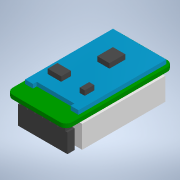
# Autodesk Inventor part: BMS
Saved by Autodesk Inventor 2020 (Build 240168000, 168)
## iProperties
Created: 2021-03-29
Part Number: BMS
Material: Generic
Document SubType Name: Modeling
Designer: Luke
Density: 1 g/cm^3
Appearance: Default
Author: Luke
Autodesk Inventor part; units mm, degrees
ref_plane "YZ Plane" through (0, 0, 0) normal (1, 0, 0) x (0, 1, 0)
ref_plane "XZ Plane" through (0, 0, 0) normal (0, 1, 0) x (-1, 0, 0)
ref_plane "XY Plane" through (0, 0, 0) normal (0, 0, 1) x (1, 0, 0)
sketch "Sketch1" plane through (0, 0, 0) normal (0, 1, 0) x (-1, 0, 0)
  line L0 (7.5, 17.125) -> (-7.5, 17.125)
  line L1 (-9.5, 15.125) -> (-9.5, -15.125)
  line L2 (-7.5, -17.125) -> (7.5, -17.125)
  line L3 (9.5, -15.125) -> (9.5, 15.125)
  line L4 (9.5, 17.125) -> (-9.5, -17.125) construction
  line L5 (-9.5, 17.125) -> (9.5, -17.125) construction
  arc A0 (7.5, -17.125) -> (9.5, -15.125) centre (7.5, -15.125) ccw
  arc A1 (-9.5, -15.125) -> (-7.5, -17.125) centre (-7.5, -15.125) ccw
  arc A2 (-7.5, 17.125) -> (-9.5, 15.125) centre (-7.5, 15.125) ccw
  arc A3 (9.5, 15.125) -> (7.5, 17.125) centre (7.5, 15.125) ccw
  point P0 (0, 0)
  dimension "d0" = 19
  dimension "d1" = 34.25
  dimension "d2" = 2
  constraints: 12 end point, 8 point on circle, 8 point on line, 8 tangent, 4 centre point, 3 equal radius, 2 midpoint, 2 parallel, 1 horizontal, 1 perpendicular
  measures "d0" distance of L5.end L4.end
  measures "d1" distance of L4.end L5.start
  measures "d2" radius of A0
extrude "Extrusion1" add sketch "Sketch1" along normal blind 1.28
sketch "Sketch2" plane through (0, 1.28, 0) normal (0, 1, 0) x (1, 0, 0)
  line L0 (8.5, -12.175) -> (8.5, 15.825)
  line L1 (8.5, 15.825) -> (-8.5, 15.825)
  line L2 (-8.5, 15.825) -> (-8.5, -12.175)
  line L3 (-8.5, -12.175) -> (8.5, 15.825) construction
  line L4 (8.5, -12.175) -> (-8.5, 15.825) construction
  line L5 (7.5, 17.125) -> (-7.5, 17.125) projected
  line L6 (0, 17.125) -> (0, 15.825)
  line L7 (-6, -10.975) -> (6, -10.975)
  line L8 (6, -10.975) -> (6, -12.175)
  line L9 (-6, -12.175) -> (-6, -10.975)
  line L10 (-8.5, -12.175) -> (-6, -12.175)
  line L11 (6, -12.175) -> (8.5, -12.175)
  point P0 (0, 0)
  point P1 (0, 15.825)
  dimension "d5" = 17
  dimension "d6" = 28
  dimension "d7" = 1.3
  dimension "d9" = 1.2
  constraints: 22 end point, 4 parallel, 3 horizontal, 3 perpendicular, 2 midpoint, 1 vertical
  measures "d5" distance of L1.end L0.end
  measures "d6" distance of L0.end L0.start
  measures "d7" distance of L6.start L6.end
  measures "d9" distance of L7.end L8.end
extrude "Extrusion2" add sketch "Sketch2" along normal blind 1.28
sketch "Sketch3" plane through (0, 0, 0) normal (0, -1, 0) x (1, 0, 0)
  line L0 (5.75, -9.895) -> (-5.75, -9.895)
  line L1 (-5.75, -9.895) -> (-5.75, 6.605)
  line L2 (-5.75, 6.605) -> (5.75, 6.605)
  line L3 (5.75, 6.605) -> (5.75, -9.895)
  line L4 (7.5, -17.125) -> (-7.5, -17.125) projected
  line L5 (0, -17.125) -> (0, -9.895)
  point P0 (0, 0)
  point P1 (0, -9.895)
  dimension "d12" = 11.5
  dimension "d13" = 16.5
  dimension "d14" = 7.23
  constraints: 10 end point, 2 midpoint, 2 parallel, 1 horizontal, 1 perpendicular, 1 vertical
  measures "d12" distance of L1.end L2.end
  measures "d13" distance of L0.end L1.end
  measures "d14" distance of L5.start L5.end
extrude "Extrusion3" add sketch "Sketch3" along normal blind 1.28
sketch "Sketch4" plane through (0, 0, 0) normal (0, -1, 0) x (1, 0, 0)
  line L0 (-7.5, 17.125) -> (7.5, 17.125) projected
  line L1 (0, 17.125) -> (0, 15.125)
  line L2 (0.2, 15.125) -> (2.24, 15.125)
  line L3 (2.44, 14.925) -> (2.44, 12.885)
  line L4 (2.24, 12.685) -> (0.2, 12.685)
  line L5 (0, 12.885) -> (0, 14.925)
  line L6 (0, 14.925) -> (0.2, 15.125)
  line L7 (2.24, 15.125) -> (2.44, 14.925)
  line L8 (2.44, 12.885) -> (2.24, 12.685)
  line L9 (0.2, 12.685) -> (0, 12.885)
  line L10 (2.64, 15.125) -> (4.68, 15.125)
  line L11 (4.88, 14.925) -> (4.88, 12.885)
  line L12 (4.68, 12.685) -> (2.64, 12.685)
  line L13 (2.44, 12.885) -> (2.44, 14.925)
  line L14 (2.44, 14.925) -> (2.64, 15.125)
  line L15 (4.68, 15.125) -> (4.88, 14.925)
  line L16 (4.88, 12.885) -> (4.68, 12.685)
  line L17 (2.64, 12.685) -> (2.44, 12.885)
  line L18 (5.08, 15.125) -> (7.12, 15.125)
  line L19 (7.32, 14.925) -> (7.32, 12.885)
  line L20 (7.12, 12.685) -> (5.08, 12.685)
  line L21 (4.88, 12.885) -> (4.88, 14.925)
  line L22 (4.88, 14.925) -> (5.08, 15.125)
  line L23 (7.12, 15.125) -> (7.32, 14.925)
  line L24 (7.32, 12.885) -> (7.12, 12.685)
  line L25 (5.08, 12.685) -> (4.88, 12.885)
  line L26 (-2.24, 15.125) -> (-0.2, 15.125)
  line L27 (0, 14.925) -> (0, 12.885)
  line L28 (-0.2, 12.685) -> (-2.24, 12.685)
  line L29 (-2.44, 12.885) -> (-2.44, 14.925)
  line L30 (-2.44, 14.925) -> (-2.24, 15.125)
  line L31 (-0.2, 15.125) -> (0, 14.925)
  line L32 (0, 12.885) -> (-0.2, 12.685)
  line L33 (-2.24, 12.685) -> (-2.44, 12.885)
  line L34 (-4.68, 15.125) -> (-2.64, 15.125)
  line L35 (-2.44, 14.925) -> (-2.44, 12.885)
  line L36 (-2.64, 12.685) -> (-4.68, 12.685)
  line L37 (-4.88, 12.885) -> (-4.88, 14.925)
  line L38 (-4.88, 14.925) -> (-4.68, 15.125)
  line L39 (-2.64, 15.125) -> (-2.44, 14.925)
  line L40 (-2.44, 12.885) -> (-2.64, 12.685)
  line L41 (-4.68, 12.685) -> (-4.88, 12.885)
  line L42 (-7.12, 15.125) -> (-5.08, 15.125)
  line L43 (-4.88, 14.925) -> (-4.88, 12.885)
  line L44 (-5.08, 12.685) -> (-7.12, 12.685)
  line L45 (-7.32, 12.885) -> (-7.32, 14.925)
  line L46 (-7.32, 14.925) -> (-7.12, 15.125)
  line L47 (-5.08, 15.125) -> (-4.88, 14.925)
  line L48 (-4.88, 12.885) -> (-5.08, 12.685)
  line L49 (-7.12, 12.685) -> (-7.32, 12.885)
  point P0 (0, 0)
  point P1 (2.44, 12.685)
  point P2 (2.44, 15.125)
  point P3 (0, 12.685)
  point P4 (2.44, 15.125)
  point P5 (4.88, 12.685)
  point P6 (4.88, 15.125)
  point P7 (2.44, 12.685)
  point P8 (4.88, 15.125)
  point P9 (7.32, 12.685)
  point P10 (7.32, 15.125)
  point P11 (4.88, 12.685)
  point P12 (-2.44, 15.125)
  point P13 (0, 12.685)
  point P14 (-2.44, 12.685)
  point P15 (-4.88, 15.125)
  point P16 (-2.44, 12.685)
  point P17 (-2.44, 15.125)
  point P18 (-4.88, 12.685)
  point P19 (-7.32, 15.125)
  point P20 (-4.88, 12.685)
  point P21 (-4.88, 15.125)
  point P22 (-7.32, 12.685)
  dimension "d27" = 2
  constraints: 98 end point, 48 point on line, 12 parallel, 6 horizontal, 6 perpendicular, 1 midpoint, 1 vertical
  measures "d27" distance of L1.start L1.end
extrude "Extrusion4" add sketch "Sketch4" along normal blind 2.44
sketch "Sketch5" plane through (0, -2.44, 0) normal (0, -1, 0) x (1, 0, 0)
  line L0 (-7.865, 15.055) -> (7.865, 15.055)
  line L1 (7.865, 15.055) -> (7.865, 12.755)
  line L2 (7.865, 12.755) -> (-7.865, 12.755)
  line L3 (-7.865, 12.755) -> (-7.865, 15.055)
  line L4 (0.2, 12.685) -> (0, 12.885) projected
  line L5 (0, 14.925) -> (0, 12.885)
  point P0 (0, 0)
  point P1 (0, 13.905)
  point P2 (0, 13.905)
  dimension "d30" = 15.73
  dimension "d31" = 2.3
  constraints: 10 end point, 2 parallel, 1 horizontal, 1 midpoint, 1 perpendicular, 1 vertical
  measures "d30" distance of L1.end L2.end
  measures "d31" distance of L0.end L1.end
extrude "Extrusion5" add sketch "Sketch5" along normal blind 6
sketch "Sketch6" plane through (0, 2.56, 0) normal (0, 1, 0) x (1, 0, 0)
  line L0 (-1.9361, 4.2441) -> (1.9639, 4.2441)
  line L1 (1.9639, 4.2441) -> (1.9639, 9.2441)
  line L2 (1.9639, 9.2441) -> (-1.9361, 9.2441)
  line L3 (-1.9361, 9.2441) -> (-1.9361, 4.2441)
  line L4 (-6.3946, -7.0839) -> (-2.0946, -7.0839)
  line L5 (-2.0946, -7.0839) -> (-2.0946, -3.9839)
  line L6 (-2.0946, -3.9839) -> (-6.3946, -3.9839)
  line L7 (-6.3946, -3.9839) -> (-6.3946, -7.0839)
  line L8 (3.9309, -7.1914) -> (5.5309, -7.1914)
  line L9 (5.5309, -7.1914) -> (5.5309, -4.1914)
  line L10 (5.5309, -4.1914) -> (3.9309, -4.1914)
  line L11 (3.9309, -4.1914) -> (3.9309, -7.1914)
  line L12 (8.5, 15.825) -> (-8.5, 15.825) projected
  point P0 (0, 0)
  point P1 (3.9309, -5.6914)
  point P2 (0, 15.825)
  point P3 (0.0139, 9.2441)
  point P4 (-2.0946, -5.5339)
  dimension "d34" = 3.9
  dimension "d35" = 5
  dimension "d36" = 4.3
  dimension "d37" = 3.1
  dimension "d38" = 1.6
  dimension "d39" = 3
  constraints: 24 end point, 6 parallel, 4 midpoint, 3 horizontal, 3 perpendicular
  measures "d34" distance of L2.end L1.end
  measures "d35" distance of L1.end L0.end
  measures "d36" distance of L6.end L5.end
  measures "d37" distance of L5.end L4.end
  measures "d38" distance of L10.end L9.end
  measures "d39" distance of L9.end L8.end
extrude "Extrusion6" add sketch "Sketch6" along normal blind 1.5
sketch "Sketch7" plane through (0, -1.28, 0) normal (0, -1, 0) x (1, 0, 0)
  line L0 (-9, 11.5) -> (9, 11.5)
  line L1 (9, 11.5) -> (9, -11.5)
  line L2 (-8.5, -11.5) -> (-9, -11.5)
  line L3 (-9, -11.5) -> (-9, 11.5)
  line L4 (-9, -11.5) -> (-9, -15)
  line L5 (-8.5, -15.825) -> (-8.5, 12.175) projected
  line L6 (-9, -11.5) -> (-5.5, -11.5) construction
  line L7 (-9, -15) -> (9, -15)
  line L8 (9, -15) -> (9, -11.5)
  dimension "d42" = 18
  dimension "d43" = 23
  dimension "d46" = 3.5
  dimension "d47" = 90
  dimension "d48" = 90
  constraints: 16 end point, 3 parallel, 3 perpendicular, 2 horizontal, 1 point on line
  measures "d42" distance of L1.end L2.end
  measures "d43" distance of L0.end L1.end
  measures "d46" distance of L2.end L4.end
  measures "d47" angle of L4 L6
  measures "d48" angle of L7 L4
ref_plane "Work Plane1" through (-19.708, -8.44, -77.2303) normal (0, 1, 0) x (0, 0, 1)
extrude "Extrusion7" add sketch "Sketch7" along normal up to surface (7.16 mm away)
body "Solid1"
